Autodesk Fusion 360 part; units mm, degrees
(part 4 of 4)
  spline S343 degree 2 poles (11.0558, -7.1187) (11.2604, -7.2715) (11.3409, -7.5484) knots 0 0 0 1 1 1
  line L153 (11.3409, -7.5484) -> (11.0803, -7.6098)
  spline S344 degree 2 poles (11.0803, -7.6098) (11.0107, -7.3915) (10.8784, -7.292) knots 0 0 0 1 1 1
  spline S345 degree 2 poles (10.8784, -7.292) (10.7461, -7.1924) (10.5455, -7.1924) knots 0 0 0 1 1 1
  spline S346 degree 2 poles (10.5455, -7.1924) (10.315, -7.1924) (10.1594, -7.3029) knots 0 0 0 1 1 1
  spline S347 degree 2 poles (10.1594, -7.3029) (10.0053, -7.4134) (9.9425, -7.6003) knots 0 0 0 1 1 1
  spline S348 degree 2 poles (9.9425, -7.6003) (9.8798, -7.7858) (9.8798, -7.9836) knots 0 0 0 1 1 1
  spline S349 degree 2 poles (9.8798, -7.9836) (9.8798, -8.2387) (9.9534, -8.4297) knots 0 0 0 1 1 1
  spline S350 degree 2 poles (9.9534, -8.4297) (10.0285, -8.6194) (10.1854, -8.7135) knots 0 0 0 1 1 1
  spline S351 degree 2 poles (3.7147, -8.854) (3.5237, -9.0355) (3.2318, -9.0355) knots 0 0 0 1 1 1
  spline S352 degree 2 poles (3.2318, -9.0355) (2.9685, -9.0355) (2.7938, -8.8786) knots 0 0 0 1 1 1
  spline S353 degree 2 poles (2.7938, -8.8786) (2.6206, -8.7217) (2.596, -8.472) knots 0 0 0 1 1 1
  line L154 (2.596, -8.472) -> (2.8416, -8.4393)
  spline S354 degree 2 poles (2.8416, -8.4393) (2.8839, -8.648) (2.9848, -8.7408) knots 0 0 0 1 1 1
  spline S355 degree 2 poles (2.9848, -8.7408) (3.0871, -8.8322) (3.2331, -8.8322) knots 0 0 0 1 1 1
  spline S356 degree 2 poles (3.2331, -8.8322) (3.4064, -8.8322) (3.5251, -8.7121) knots 0 0 0 1 1 1
  spline S357 degree 2 poles (3.5251, -8.7121) (3.6451, -8.5921) (3.6451, -8.4147) knots 0 0 0 1 1 1
  spline S358 degree 2 poles (3.6451, -8.4147) (3.6451, -8.2456) (3.5346, -8.1364) knots 0 0 0 1 1 1
  spline S359 degree 2 poles (3.5346, -8.1364) (3.4241, -8.0259) (3.2536, -8.0259) knots 0 0 0 1 1 1
  spline S360 degree 2 poles (3.2536, -8.0259) (3.184, -8.0259) (3.0803, -8.0532) knots 0 0 0 1 1 1
  line L155 (3.0803, -8.0532) -> (3.1076, -7.8377)
  spline S361 degree 2 poles (3.1076, -7.8377) (3.1322, -7.8404) (3.1472, -7.8404) knots 0 0 0 1 1 1
  spline S362 degree 2 poles (3.1472, -7.8404) (3.3041, -7.8404) (3.4296, -7.7585) knots 0 0 0 1 1 1
  spline S363 degree 2 poles (3.4296, -7.7585) (3.5551, -7.6767) (3.5551, -7.5061) knots 0 0 0 1 1 1
  spline S364 degree 2 poles (3.5551, -7.5061) (3.5551, -7.3711) (3.4637, -7.2824) knots 0 0 0 1 1 1
  spline S365 degree 2 poles (3.4637, -7.2824) (3.3723, -7.1937) (3.2277, -7.1937) knots 0 0 0 1 1 1
  spline S366 degree 2 poles (3.2277, -7.1937) (3.0844, -7.1937) (2.9889, -7.2838) knots 0 0 0 1 1 1
  spline S367 degree 2 poles (2.9889, -7.2838) (2.8934, -7.3738) (2.8661, -7.5539) knots 0 0 0 1 1 1
  line L156 (2.8661, -7.5539) -> (2.6206, -7.5102)
  spline S368 degree 2 poles (2.6206, -7.5102) (2.6656, -7.2633) (2.8252, -7.1282) knots 0 0 0 1 1 1
  spline S369 degree 2 poles (2.8252, -7.1282) (2.9848, -6.9918) (3.2222, -6.9918) knots 0 0 0 1 1 1
  spline S370 degree 2 poles (3.2222, -6.9918) (3.3859, -6.9918) (3.5237, -7.0628) knots 0 0 0 1 1 1
  spline S371 degree 2 poles (3.5237, -7.0628) (3.6615, -7.1323) (3.7338, -7.2538) knots 0 0 0 1 1 1
  spline S372 degree 2 poles (3.7338, -7.2538) (3.8075, -7.3752) (3.8075, -7.5116) knots 0 0 0 1 1 1
  spline S373 degree 2 poles (3.8075, -7.5116) (3.8075, -7.6412) (3.7379, -7.7476) knots 0 0 0 1 1 1
  spline S374 degree 2 poles (3.7379, -7.7476) (3.6683, -7.854) (3.5319, -7.9168) knots 0 0 0 1 1 1
  spline S375 degree 2 poles (3.5319, -7.9168) (3.7092, -7.9577) (3.8075, -8.0873) knots 0 0 0 1 1 1
  spline S376 degree 2 poles (3.8075, -8.0873) (3.9057, -8.2156) (3.9057, -8.4093) knots 0 0 0 1 1 1
  spline S377 degree 2 poles (3.9057, -8.4093) (3.9057, -8.6712) (3.7147, -8.854) knots 0 0 0 1 1 1
  line L157 (-0.0141, -2.5211) -> (-0.2842, -2.5211)
  line L158 (-0.2842, -2.5211) -> (-0.2842, -3)
  line L159 (-0.2842, -3) -> (-0.5298, -3)
  line L160 (-0.5298, -3) -> (-0.5298, -2.5211)
  line L161 (-0.5298, -2.5211) -> (-1.3975, -2.5211)
  line L162 (-1.3975, -2.5211) -> (-1.3975, -2.296)
  line L163 (-1.3975, -2.296) -> (-0.4848, -1)
  line L164 (-0.4848, -1) -> (-0.2842, -1)
  line L165 (-0.2842, -1) -> (-0.2842, -2.296)
  line L166 (-0.2842, -2.296) -> (-0.0141, -2.296)
  line L167 (-0.0141, -2.296) -> (-0.0141, -2.5211)
  line L168 (-5.8463, -2.1528) -> (-5.0919, -2.1528)
  line L169 (-5.0919, -2.1528) -> (-5.0919, -2.3997)
  line L170 (-5.0919, -2.3997) -> (-5.8463, -2.3997)
  line L171 (-5.8463, -2.3997) -> (-5.8463, -2.1528)
  spline S378 degree 2 poles (-2.3822, -4.2592) (-2.228, -4.1214) (-2.1639, -3.9918) knots 0 0 0 1 1 1
  line L172 (-2.1639, -3.9918) -> (-2.0056, -3.9918)
  line L173 (-2.0056, -3.9918) -> (-2.0056, -6)
  line L174 (-2.0056, -6) -> (-2.2512, -6)
  line L175 (-2.2512, -6) -> (-2.2512, -4.4352)
  spline S379 degree 2 poles (-2.2512, -4.4352) (-2.3399, -4.5198) (-2.4845, -4.6044) knots 0 0 0 1 1 1
  spline S380 degree 2 poles (-2.4845, -4.6044) (-2.6277, -4.6889) (-2.7423, -4.7312) knots 0 0 0 1 1 1
  line L176 (-2.7423, -4.7312) -> (-2.7423, -4.4939)
  spline S381 degree 2 poles (-2.7423, -4.4939) (-2.5363, -4.397) (-2.3822, -4.2592) knots 0 0 0 1 1 1
  spline S382 degree 2 poles (-4.2457, -5.9168) (-4.389, -6.0341) (-4.6086, -6.0341) knots 0 0 0 1 1 1
  spline S383 degree 2 poles (-4.6086, -6.0341) (-4.8979, -6.0341) (-5.0629, -5.8267) knots 0 0 0 1 1 1
  spline S384 degree 2 poles (-5.0629, -5.8267) (-5.2607, -5.5771) (-5.2607, -5.0136) knots 0 0 0 1 1 1
  spline S385 degree 2 poles (-5.2607, -5.0136) (-5.2607, -4.6589) (-5.1884, -4.4434) knots 0 0 0 1 1 1
  spline S386 degree 2 poles (-5.1884, -4.4434) (-5.1148, -4.2265) (-4.9715, -4.1091) knots 0 0 0 1 1 1
  spline S387 degree 2 poles (-4.9715, -4.1091) (-4.8269, -3.9918) (-4.6086, -3.9918) knots 0 0 0 1 1 1
  spline S388 degree 2 poles (-4.6086, -3.9918) (-4.4476, -3.9918) (-4.3262, -4.0573) knots 0 0 0 1 1 1
  spline S389 degree 2 poles (-4.3262, -4.0573) (-4.2048, -4.1214) (-4.1257, -4.2442) knots 0 0 0 1 1 1
  spline S390 degree 2 poles (-4.1257, -4.2442) (-4.0466, -4.3656) (-4.0015, -4.5416) knots 0 0 0 1 1 1
  spline S391 degree 2 poles (-4.0015, -4.5416) (-3.9565, -4.7162) (-3.9565, -5.0136) knots 0 0 0 1 1 1
  spline S392 degree 2 poles (-3.9565, -5.0136) (-3.9565, -5.3656) (-4.0288, -5.5825) knots 0 0 0 1 1 1
  spline S393 degree 2 poles (-4.0288, -5.5825) (-4.1011, -5.7981) (-4.2457, -5.9168) knots 0 0 0 1 1 1
  spline S394 degree 2 poles (-7.3165, -0.0412) (-7.4213, -0.1198) (-7.5801, -0.1607) knots 0 0 0 1 1 1
  spline S395 degree 2 poles (-7.5801, -0.1607) (-7.7373, -0.2) (-7.9665, -0.2) knots 0 0 0 1 1 1
  line L177 (-7.9665, -0.2) -> (-8.8816, -0.2)
  line L178 (-8.8816, -0.2) -> (-8.8816, 2.2)
  line L179 (-8.8816, 2.2) -> (-7.9812, 2.2)
  spline S396 degree 2 poles (-7.9812, 2.2) (-7.7062, 2.2) (-7.5408, 2.1263) knots 0 0 0 1 1 1
  spline S397 degree 2 poles (-7.5408, 2.1263) (-7.3738, 2.0543) (-7.2805, 1.902) knots 0 0 0 1 1 1
  spline S398 degree 2 poles (-7.2805, 1.902) (-7.1856, 1.7514) (-7.1856, 1.5861) knots 0 0 0 1 1 1
  spline S399 degree 2 poles (-7.1856, 1.5861) (-7.1856, 1.4322) (-7.2691, 1.2963) knots 0 0 0 1 1 1
  spline S400 degree 2 poles (-7.2691, 1.2963) (-7.3526, 1.1604) (-7.5212, 1.0769) knots 0 0 0 1 1 1
  spline S401 degree 2 poles (-7.5212, 1.0769) (-7.3035, 1.0131) (-7.1872, 0.8592) knots 0 0 0 1 1 1
  spline S402 degree 2 poles (-7.1872, 0.8592) (-7.0693, 0.7053) (-7.0693, 0.4958) knots 0 0 0 1 1 1
  spline S403 degree 2 poles (-7.0693, 0.4958) (-7.0693, 0.3271) (-7.1414, 0.1814) knots 0 0 0 1 1 1
  spline S404 degree 2 poles (-7.1414, 0.1814) (-7.2118, 0.0374) (-7.3165, -0.0412) knots 0 0 0 1 1 1
  spline S405 degree 2 poles (-10.9718, -6.0341) (-11.2433, -6.0341) (-11.4275, -5.955) knots 0 0 0 1 1 1
  spline S406 degree 2 poles (-11.4275, -5.955) (-11.6103, -5.8759) (-11.7153, -5.7176) knots 0 0 0 1 1 1
  spline S407 degree 2 poles (-11.7153, -5.7176) (-11.819, -5.558) (-11.8245, -5.3574) knots 0 0 0 1 1 1
  line L180 (-11.8245, -5.3574) -> (-11.5748, -5.3356)
  spline S408 degree 2 poles (-11.5748, -5.3356) (-11.5571, -5.4857) (-11.493, -5.5825) knots 0 0 0 1 1 1
  spline S409 degree 2 poles (-11.493, -5.5825) (-11.4275, -5.678) (-11.2911, -5.7381) knots 0 0 0 1 1 1
  spline S410 degree 2 poles (-11.2911, -5.7381) (-11.1546, -5.7967) (-10.9841, -5.7967) knots 0 0 0 1 1 1
  spline S411 degree 2 poles (-10.9841, -5.7967) (-10.8327, -5.7967) (-10.7167, -5.7517) knots 0 0 0 1 1 1
  spline S412 degree 2 poles (-10.7167, -5.7517) (-10.6008, -5.7067) (-10.5448, -5.6289) knots 0 0 0 1 1 1
  spline S413 degree 2 poles (-10.5448, -5.6289) (-10.4875, -5.5498) (-10.4875, -5.457) knots 0 0 0 1 1 1
  spline S414 degree 2 poles (-10.4875, -5.457) (-10.4875, -5.3629) (-10.5421, -5.2933) knots 0 0 0 1 1 1
  spline S415 degree 2 poles (-10.5421, -5.2933) (-10.5967, -5.2224) (-10.7222, -5.1746) knots 0 0 0 1 1 1
  spline S416 degree 2 poles (-10.7222, -5.1746) (-10.8027, -5.1432) (-11.0782, -5.0778) knots 0 0 0 1 1 1
  spline S417 degree 2 poles (-11.0782, -5.0778) (-11.3538, -5.0109) (-11.4643, -4.9523) knots 0 0 0 1 1 1
  spline S418 degree 2 poles (-11.4643, -4.9523) (-11.6076, -4.8772) (-11.6785, -4.7667) knots 0 0 0 1 1 1
  spline S419 degree 2 poles (-11.6785, -4.7667) (-11.7481, -4.6548) (-11.7481, -4.5171) knots 0 0 0 1 1 1
  spline S420 degree 2 poles (-11.7481, -4.5171) (-11.7481, -4.3656) (-11.6621, -4.2347) knots 0 0 0 1 1 1
  spline S421 degree 2 poles (-11.6621, -4.2347) (-11.5762, -4.1023) (-11.4111, -4.0341) knots 0 0 0 1 1 1
  spline S422 degree 2 poles (-11.4111, -4.0341) (-11.246, -3.9659) (-11.0441, -3.9659) knots 0 0 0 1 1 1
  spline S423 degree 2 poles (-11.0441, -3.9659) (-10.8218, -3.9659) (-10.6526, -4.0382) knots 0 0 0 1 1 1
  spline S424 degree 2 poles (-10.6526, -4.0382) (-10.4821, -4.1091) (-10.3907, -4.2483) knots 0 0 0 1 1 1
  spline S425 degree 2 poles (-10.3907, -4.2483) (-10.2993, -4.3874) (-10.2924, -4.5634) knots 0 0 0 1 1 1
  line L181 (-10.2924, -4.5634) -> (-10.5462, -4.5825)
  spline S426 degree 2 poles (-10.5462, -4.5825) (-10.5666, -4.3929) (-10.6853, -4.296) knots 0 0 0 1 1 1
  spline S427 degree 2 poles (-10.6853, -4.296) (-10.8027, -4.1992) (-11.0332, -4.1992) knots 0 0 0 1 1 1
  spline S428 degree 2 poles (-11.0332, -4.1992) (-11.2733, -4.1992) (-11.3838, -4.2879) knots 0 0 0 1 1 1
  spline S429 degree 2 poles (-11.3838, -4.2879) (-11.493, -4.3752) (-11.493, -4.4993) knots 0 0 0 1 1 1
  spline S430 degree 2 poles (-11.493, -4.4993) (-11.493, -4.6071) (-11.4152, -4.6767) knots 0 0 0 1 1 1
  spline S431 degree 2 poles (-11.4152, -4.6767) (-11.3388, -4.7462) (-11.0168, -4.8199) knots 0 0 0 1 1 1
  spline S432 degree 2 poles (-11.0168, -4.8199) (-10.6935, -4.8922) (-10.5735, -4.9468) knots 0 0 0 1 1 1
  spline S433 degree 2 poles (-10.5735, -4.9468) (-10.3988, -5.0273) (-10.3156, -5.1514) knots 0 0 0 1 1 1
  spline S434 degree 2 poles (-10.3156, -5.1514) (-10.2324, -5.2742) (-10.2324, -5.4352) knots 0 0 0 1 1 1
  spline S435 degree 2 poles (-10.2324, -5.4352) (-10.2324, -5.5948) (-10.3238, -5.7367) knots 0 0 0 1 1 1
  spline S436 degree 2 poles (-10.3238, -5.7367) (-10.4152, -5.8772) (-10.5871, -5.9563) knots 0 0 0 1 1 1
  spline S437 degree 2 poles (-10.5871, -5.9563) (-10.7576, -6.0341) (-10.9718, -6.0341) knots 0 0 0 1 1 1
  line L182 (-7.1267, -8.1869) -> (-7.6397, -8.1869)
  line L183 (-7.6397, -8.1869) -> (-7.6397, -9)
  line L184 (-7.6397, -9) -> (-7.9043, -9)
  line L185 (-7.9043, -9) -> (-7.9043, -7)
  line L186 (-7.9043, -7) -> (-7.1499, -7)
  spline S438 degree 2 poles (-7.1499, -7) (-6.9507, -7) (-6.8457, -7.0191) knots 0 0 0 1 1 1
  spline S439 degree 2 poles (-6.8457, -7.0191) (-6.6983, -7.0437) (-6.5987, -7.1132) knots 0 0 0 1 1 1
  spline S440 degree 2 poles (-6.5987, -7.1132) (-6.4991, -7.1814) (-6.4391, -7.3056) knots 0 0 0 1 1 1
  spline S441 degree 2 poles (-6.4391, -7.3056) (-6.3777, -7.4297) (-6.3777, -7.5784) knots 0 0 0 1 1 1
  spline S442 degree 2 poles (-6.3777, -7.5784) (-6.3777, -7.8336) (-6.5401, -8.0109) knots 0 0 0 1 1 1
  spline S443 degree 2 poles (-6.5401, -8.0109) (-6.7024, -8.1869) (-7.1267, -8.1869) knots 0 0 0 1 1 1
  spline S444 degree 2 poles (-8.7686, -4.2415) (-8.7999, -4.3793) (-8.8272, -4.4761) knots 0 0 0 1 1 1
  line L187 (-8.8272, -4.4761) -> (-9.2515, -6)
  line L188 (-9.2515, -6) -> (-9.5216, -6)
  line L189 (-9.5216, -6) -> (-10.0523, -4)
  line L190 (-10.0523, -4) -> (-9.7808, -4)
  line L191 (-9.7808, -4) -> (-9.4766, -5.3111)
  spline S445 degree 2 poles (-9.4766, -5.3111) (-9.4275, -5.5171) (-9.392, -5.7203) knots 0 0 0 1 1 1
  spline S446 degree 2 poles (-9.392, -5.7203) (-9.3156, -5.3997) (-9.302, -5.3506) knots 0 0 0 1 1 1
  line L192 (-9.302, -5.3506) -> (-8.9214, -4)
  line L193 (-8.9214, -4) -> (-8.6021, -4)
  line L194 (-8.6021, -4) -> (-8.3156, -5.0123)
  spline S447 degree 2 poles (-8.3156, -5.0123) (-8.2078, -5.3888) (-8.1601, -5.7203) knots 0 0 0 1 1 1
  spline S448 degree 2 poles (-8.1601, -5.7203) (-8.1219, -5.5307) (-8.0605, -5.2851) knots 0 0 0 1 1 1
  line L195 (-8.0605, -5.2851) -> (-7.7467, -4)
  line L196 (-7.7467, -4) -> (-7.4807, -4)
  line L197 (-7.4807, -4) -> (-8.0291, -6)
  line L198 (-8.0291, -6) -> (-8.2842, -6)
  line L199 (-8.2842, -6) -> (-8.7058, -4.4761)
  spline S449 degree 2 poles (-8.7058, -4.4761) (-8.759, -4.2851) (-8.7686, -4.2415) knots 0 0 0 1 1 1
  line L200 (-9.8845, -2.1528) -> (-9.1301, -2.1528)
  line L201 (-9.1301, -2.1528) -> (-9.1301, -2.3997)
  line L202 (-9.1301, -2.3997) -> (-9.8845, -2.3997)
  line L203 (-9.8845, -2.3997) -> (-9.8845, -2.1528)
  line L204 (-3.5691, -5.7203) -> (-3.2894, -5.7203)
  line L205 (-3.2894, -5.7203) -> (-3.2894, -6)
  line L206 (-3.2894, -6) -> (-3.5691, -6)
  line L207 (-3.5691, -6) -> (-3.5691, -5.7203)
  line L208 (-0.1598, -5.3943) -> (-0.9961, -5.3943)
  line L209 (-0.9961, -5.3943) -> (-1.2157, -6)
  line L210 (-1.2157, -6) -> (-1.4968, -6)
  line L211 (-1.4968, -6) -> (-0.7287, -4)
  line L212 (-0.7287, -4) -> (-0.4436, -4)
  line L213 (-0.4436, -4) -> (0.375, -6)
  line L214 (0.375, -6) -> (0.0735, -6)
  line L215 (0.0735, -6) -> (-0.1598, -5.3943)
  spline S450 degree 2 poles (-5.4656, -0.2409) (-5.7914, -0.2409) (-6.0124, -0.146) knots 0 0 0 1 1 1
  spline S451 degree 2 poles (-6.0124, -0.146) (-6.2318, -0.051) (-6.3579, 0.1389) knots 0 0 0 1 1 1
  spline S452 degree 2 poles (-6.3579, 0.1389) (-6.4823, 0.3304) (-6.4888, 0.5711) knots 0 0 0 1 1 1
  line L216 (-6.4888, 0.5711) -> (-6.1892, 0.5973)
  spline S453 degree 2 poles (-6.1892, 0.5973) (-6.168, 0.4172) (-6.091, 0.301) knots 0 0 0 1 1 1
  spline S454 degree 2 poles (-6.091, 0.301) (-6.0124, 0.1864) (-5.8487, 0.1143) knots 0 0 0 1 1 1
  spline S455 degree 2 poles (-5.8487, 0.1143) (-5.685, 0.0439) (-5.4804, 0.0439) knots 0 0 0 1 1 1
  spline S456 degree 2 poles (-5.4804, 0.0439) (-5.2987, 0.0439) (-5.1595, 0.098) knots 0 0 0 1 1 1
  spline S457 degree 2 poles (-5.1595, 0.098) (-5.0203, 0.152) (-4.9532, 0.2453) knots 0 0 0 1 1 1
  spline S458 degree 2 poles (-4.9532, 0.2453) (-4.8845, 0.3402) (-4.8845, 0.4516) knots 0 0 0 1 1 1
  spline S459 degree 2 poles (-4.8845, 0.4516) (-4.8845, 0.5645) (-4.9499, 0.648) knots 0 0 0 1 1 1
  spline S460 degree 2 poles (-4.9499, 0.648) (-5.0154, 0.7332) (-5.166, 0.7905) knots 0 0 0 1 1 1
  spline S461 degree 2 poles (-5.166, 0.7905) (-5.2626, 0.8281) (-5.5933, 0.9067) knots 0 0 0 1 1 1
  spline S462 degree 2 poles (-5.5933, 0.9067) (-5.924, 0.9869) (-6.0566, 1.0573) knots 0 0 0 1 1 1
  spline S463 degree 2 poles (-6.0566, 1.0573) (-6.2285, 1.1473) (-6.3137, 1.2799) knots 0 0 0 1 1 1
  spline S464 degree 2 poles (-6.3137, 1.2799) (-6.3971, 1.4142) (-6.3971, 1.5795) knots 0 0 0 1 1 1
  spline S465 degree 2 poles (-6.3971, 1.5795) (-6.3971, 1.7613) (-6.294, 1.9184) knots 0 0 0 1 1 1
  spline S466 degree 2 poles (-6.294, 1.9184) (-6.1909, 2.0772) (-5.9928, 2.1591) knots 0 0 0 1 1 1
  spline S467 degree 2 poles (-5.9928, 2.1591) (-5.7947, 2.2409) (-5.5524, 2.2409) knots 0 0 0 1 1 1
  spline S468 degree 2 poles (-5.5524, 2.2409) (-5.2856, 2.2409) (-5.0826, 2.1542) knots 0 0 0 1 1 1
  spline S469 degree 2 poles (-5.0826, 2.1542) (-4.8779, 2.069) (-4.7682, 1.902) knots 0 0 0 1 1 1
  spline S470 degree 2 poles (-4.7682, 1.902) (-4.6585, 1.7351) (-4.6504, 1.5239) knots 0 0 0 1 1 1
  line L217 (-4.6504, 1.5239) -> (-4.9549, 1.501)
  spline S471 degree 2 poles (-4.9549, 1.501) (-4.9794, 1.7285) (-5.1218, 1.8447) knots 0 0 0 1 1 1
  spline S472 degree 2 poles (-5.1218, 1.8447) (-5.2626, 1.961) (-5.5393, 1.961) knots 0 0 0 1 1 1
  spline S473 degree 2 poles (-5.5393, 1.961) (-5.8274, 1.961) (-5.96, 1.8546) knots 0 0 0 1 1 1
  spline S474 degree 2 poles (-5.96, 1.8546) (-6.091, 1.7498) (-6.091, 1.6008) knots 0 0 0 1 1 1
  spline S475 degree 2 poles (-6.091, 1.6008) (-6.091, 1.4715) (-5.9977, 1.388) knots 0 0 0 1 1 1
  spline S476 degree 2 poles (-5.9977, 1.388) (-5.906, 1.3045) (-5.5197, 1.2161) knots 0 0 0 1 1 1
  spline S477 degree 2 poles (-5.5197, 1.2161) (-5.1317, 1.1293) (-4.9876, 1.0638) knots 0 0 0 1 1 1
  spline S478 degree 2 poles (-4.9876, 1.0638) (-4.778, 0.9673) (-4.6782, 0.8183) knots 0 0 0 1 1 1
  spline S479 degree 2 poles (-4.6782, 0.8183) (-4.5783, 0.6709) (-4.5783, 0.4778) knots 0 0 0 1 1 1
  spline S480 degree 2 poles (-4.5783, 0.4778) (-4.5783, 0.2862) (-4.688, 0.116) knots 0 0 0 1 1 1
  spline S481 degree 2 poles (-4.688, 0.116) (-4.7977, -0.0527) (-5.004, -0.1476) knots 0 0 0 1 1 1
  spline S482 degree 2 poles (-5.004, -0.1476) (-5.2086, -0.2409) (-5.4656, -0.2409) knots 0 0 0 1 1 1
  line L218 (7.1581, -4) -> (7.4282, -4)
  line L219 (7.4282, -4) -> (6.6451, -6)
  line L220 (6.6451, -6) -> (6.3736, -6)
  line L221 (6.3736, -6) -> (5.5987, -4)
  line L222 (5.5987, -4) -> (5.8852, -4)
  line L223 (5.8852, -4) -> (6.405, -5.4529)
  spline S483 degree 2 poles (6.405, -5.4529) (6.4678, -5.6276) (6.5101, -5.7804) knots 0 0 0 1 1 1
  spline S484 degree 2 poles (6.5101, -5.7804) (6.5564, -5.6166) (6.6178, -5.4529) knots 0 0 0 1 1 1
  line L224 (6.6178, -5.4529) -> (7.1581, -4)
  spline S485 degree 2 poles (5.1635, -8.9168) (5.0203, -9.0341) (4.8006, -9.0341) knots 0 0 0 1 1 1
  spline S486 degree 2 poles (4.8006, -9.0341) (4.5114, -9.0341) (4.3464, -8.8267) knots 0 0 0 1 1 1
  spline S487 degree 2 poles (4.3464, -8.8267) (4.1485, -8.5771) (4.1485, -8.0136) knots 0 0 0 1 1 1
  spline S488 degree 2 poles (4.1485, -8.0136) (4.1485, -7.6589) (4.2208, -7.4434) knots 0 0 0 1 1 1
  spline S489 degree 2 poles (4.2208, -7.4434) (4.2945, -7.2265) (4.4378, -7.1091) knots 0 0 0 1 1 1
  spline S490 degree 2 poles (4.4378, -7.1091) (4.5824, -6.9918) (4.8006, -6.9918) knots 0 0 0 1 1 1
  spline S491 degree 2 poles (4.8006, -6.9918) (4.9616, -6.9918) (5.083, -7.0573) knots 0 0 0 1 1 1
  spline S492 degree 2 poles (5.083, -7.0573) (5.2045, -7.1214) (5.2836, -7.2442) knots 0 0 0 1 1 1
  spline S493 degree 2 poles (5.2836, -7.2442) (5.3627, -7.3656) (5.4077, -7.5416) knots 0 0 0 1 1 1
  spline S494 degree 2 poles (5.4077, -7.5416) (5.4528, -7.7162) (5.4528, -8.0136) knots 0 0 0 1 1 1
  spline S495 degree 2 poles (5.4528, -8.0136) (5.4528, -8.3656) (5.3805, -8.5825) knots 0 0 0 1 1 1
  spline S496 degree 2 poles (5.3805, -8.5825) (5.3082, -8.7981) (5.1635, -8.9168) knots 0 0 0 1 1 1
  spline S497 degree 2 poles (10.1854, -5.7135) (10.3423, -5.8076) (10.5251, -5.8076) knots 0 0 0 1 1 1
  spline S498 degree 2 poles (10.5251, -5.8076) (10.7474, -5.8076) (10.9016, -5.6794) knots 0 0 0 1 1 1
  spline S499 degree 2 poles (10.9016, -5.6794) (11.0558, -5.5512) (11.1103, -5.2988) knots 0 0 0 1 1 1
  line L225 (11.1103, -5.2988) -> (11.375, -5.3656)
  spline S500 degree 2 poles (11.375, -5.3656) (11.2918, -5.6917) (11.0749, -5.8636) knots 0 0 0 1 1 1
  spline S501 degree 2 poles (11.0749, -5.8636) (10.8593, -6.0341) (10.5469, -6.0341) knots 0 0 0 1 1 1
  spline S502 degree 2 poles (10.5469, -6.0341) (10.2236, -6.0341) (10.0203, -5.9031) knots 0 0 0 1 1 1
  spline S503 degree 2 poles (10.0203, -5.9031) (9.8184, -5.7708) (9.712, -5.5211) knots 0 0 0 1 1 1
  spline S504 degree 2 poles (9.712, -5.5211) (9.6069, -5.2715) (9.6069, -4.985) knots 0 0 0 1 1 1
  spline S505 degree 2 poles (9.6069, -4.985) (9.6069, -4.6726) (9.7256, -4.4407) knots 0 0 0 1 1 1
  spline S506 degree 2 poles (9.7256, -4.4407) (9.8457, -4.2074) (10.0653, -4.0873) knots 0 0 0 1 1 1
  spline S507 degree 2 poles (10.0653, -4.0873) (10.2863, -3.9659) (10.551, -3.9659) knots 0 0 0 1 1 1
  spline S508 degree 2 poles (10.551, -3.9659) (10.8511, -3.9659) (11.0558, -4.1187) knots 0 0 0 1 1 1
  spline S509 degree 2 poles (11.0558, -4.1187) (11.2604, -4.2715) (11.3409, -4.5484) knots 0 0 0 1 1 1
  line L226 (11.3409, -4.5484) -> (11.0803, -4.6098)
  spline S510 degree 2 poles (11.0803, -4.6098) (11.0107, -4.3915) (10.8784, -4.292) knots 0 0 0 1 1 1
  spline S511 degree 2 poles (10.8784, -4.292) (10.7461, -4.1924) (10.5455, -4.1924) knots 0 0 0 1 1 1
  spline S512 degree 2 poles (10.5455, -4.1924) (10.315, -4.1924) (10.1594, -4.3029) knots 0 0 0 1 1 1
  spline S513 degree 2 poles (10.1594, -4.3029) (10.0053, -4.4134) (9.9425, -4.6003) knots 0 0 0 1 1 1
  spline S514 degree 2 poles (9.9425, -4.6003) (9.8798, -4.7858) (9.8798, -4.9836) knots 0 0 0 1 1 1
  spline S515 degree 2 poles (9.8798, -4.9836) (9.8798, -5.2387) (9.9534, -5.4297) knots 0 0 0 1 1 1
  spline S516 degree 2 poles (9.9534, -5.4297) (10.0285, -5.6194) (10.1854, -5.7135) knots 0 0 0 1 1 1
  spline S517 degree 2 poles (6.5275, -1.2592) (6.6816, -1.1214) (6.7458, -0.9918) knots 0 0 0 1 1 1
  line L227 (6.7458, -0.9918) -> (6.904, -0.9918)
  line L228 (6.904, -0.9918) -> (6.904, -3)
  line L229 (6.904, -3) -> (6.6585, -3)
  line L230 (6.6585, -3) -> (6.6585, -1.4352)
  spline S518 degree 2 poles (6.6585, -1.4352) (6.5698, -1.5198) (6.4252, -1.6044) knots 0 0 0 1 1 1
  spline S519 degree 2 poles (6.4252, -1.6044) (6.2819, -1.6889) (6.1673, -1.7312) knots 0 0 0 1 1 1
  line L231 (6.1673, -1.7312) -> (6.1673, -1.4939)
  spline S520 degree 2 poles (6.1673, -1.4939) (6.3733, -1.397) (6.5275, -1.2592) knots 0 0 0 1 1 1
  line L232 (0.2096, -2.1528) -> (0.964, -2.1528)
  line L233 (0.964, -2.1528) -> (0.964, -2.3997)
  line L234 (0.964, -2.3997) -> (0.2096, -2.3997)
  line L235 (0.2096, -2.3997) -> (0.2096, -2.1528)
  spline S521 degree 2 poles (7.7779, 1.8889) (7.9629, 2.0543) (8.0398, 2.2098) knots 0 0 0 1 1 1
  line L236 (8.0398, 2.2098) -> (8.2298, 2.2098)
  line L237 (8.2298, 2.2098) -> (8.2298, -0.2)
  line L238 (8.2298, -0.2) -> (7.9351, -0.2)
  line L239 (7.9351, -0.2) -> (7.9351, 1.6778)
  spline S522 degree 2 poles (7.9351, 1.6778) (7.8287, 1.5763) (7.6551, 1.4748) knots 0 0 0 1 1 1
  spline S523 degree 2 poles (7.6551, 1.4748) (7.4832, 1.3733) (7.3457, 1.3225) knots 0 0 0 1 1 1
  line L240 (7.3457, 1.3225) -> (7.3457, 1.6074)
  spline S524 degree 2 poles (7.3457, 1.6074) (7.5929, 1.7236) (7.7779, 1.8889) knots 0 0 0 1 1 1
  spline S525 degree 2 poles (-9.2484, 3.3595) (-9.3917, 3.2234) (-9.6106, 3.2234) knots 0 0 0 1 1 1
  spline S526 degree 2 poles (-9.6106, 3.2234) (-9.8081, 3.2234) (-9.9391, 3.3411) knots 0 0 0 1 1 1
  spline S527 degree 2 poles (-9.9391, 3.3411) (-10.069, 3.4587) (-10.0875, 3.646) knots 0 0 0 1 1 1
  line L241 (-10.0875, 3.646) -> (-9.9033, 3.6705)
  spline S528 degree 2 poles (-9.9033, 3.6705) (-9.8716, 3.514) (-9.7958, 3.4444) knots 0 0 0 1 1 1
  spline S529 degree 2 poles (-9.7958, 3.4444) (-9.7191, 3.3759) (-9.6096, 3.3759) knots 0 0 0 1 1 1
  spline S530 degree 2 poles (-9.6096, 3.3759) (-9.4797, 3.3759) (-9.3907, 3.4659) knots 0 0 0 1 1 1
  spline S531 degree 2 poles (-9.3907, 3.4659) (-9.3006, 3.5559) (-9.3006, 3.6889) knots 0 0 0 1 1 1
  spline S532 degree 2 poles (-9.3006, 3.6889) (-9.3006, 3.8158) (-9.3835, 3.8977) knots 0 0 0 1 1 1
  spline S533 degree 2 poles (-9.3835, 3.8977) (-9.4664, 3.9806) (-9.5943, 3.9806) knots 0 0 0 1 1 1
  spline S534 degree 2 poles (-9.5943, 3.9806) (-9.6465, 3.9806) (-9.7242, 3.9601) knots 0 0 0 1 1 1
  line L242 (-9.7242, 3.9601) -> (-9.7038, 4.1218)
  spline S535 degree 2 poles (-9.7038, 4.1218) (-9.6853, 4.1197) (-9.6741, 4.1197) knots 0 0 0 1 1 1
  spline S536 degree 2 poles (-9.6741, 4.1197) (-9.5564, 4.1197) (-9.4623, 4.1811) knots 0 0 0 1 1 1
  spline S537 degree 2 poles (-9.4623, 4.1811) (-9.3681, 4.2425) (-9.3681, 4.3704) knots 0 0 0 1 1 1
  spline S538 degree 2 poles (-9.3681, 4.3704) (-9.3681, 4.4717) (-9.4367, 4.5382) knots 0 0 0 1 1 1
  spline S539 degree 2 poles (-9.4367, 4.5382) (-9.5053, 4.6047) (-9.6137, 4.6047) knots 0 0 0 1 1 1
  spline S540 degree 2 poles (-9.6137, 4.6047) (-9.7211, 4.6047) (-9.7928, 4.5372) knots 0 0 0 1 1 1
  spline S541 degree 2 poles (-9.7928, 4.5372) (-9.8644, 4.4696) (-9.8849, 4.3346) knots 0 0 0 1 1 1
  line L243 (-9.8849, 4.3346) -> (-10.069, 4.3673)
  spline S542 degree 2 poles (-10.069, 4.3673) (-10.0353, 4.5525) (-9.9156, 4.6538) knots 0 0 0 1 1 1
  spline S543 degree 2 poles (-9.9156, 4.6538) (-9.7958, 4.7561) (-9.6178, 4.7561) knots 0 0 0 1 1 1
  spline S544 degree 2 poles (-9.6178, 4.7561) (-9.495, 4.7561) (-9.3917, 4.7029) knots 0 0 0 1 1 1
  spline S545 degree 2 poles (-9.3917, 4.7029) (-9.2883, 4.6508) (-9.2341, 4.5597) knots 0 0 0 1 1 1
  spline S546 degree 2 poles (-9.2341, 4.5597) (-9.1789, 4.4686) (-9.1789, 4.3663) knots 0 0 0 1 1 1
  spline S547 degree 2 poles (-9.1789, 4.3663) (-9.1789, 4.2691) (-9.231, 4.1893) knots 0 0 0 1 1 1
  spline S548 degree 2 poles (-9.231, 4.1893) (-9.2832, 4.1095) (-9.3855, 4.0624) knots 0 0 0 1 1 1
  spline S549 degree 2 poles (-9.3855, 4.0624) (-9.2525, 4.0317) (-9.1789, 3.9345) knots 0 0 0 1 1 1
  spline S550 degree 2 poles (-9.1789, 3.9345) (-9.1052, 3.8383) (-9.1052, 3.693) knots 0 0 0 1 1 1
  spline S551 degree 2 poles (-9.1052, 3.693) (-9.1052, 3.4966) (-9.2484, 3.3595) knots 0 0 0 1 1 1
  line L244 (-4.0281, 3.25) -> (-4.816, 4.4287)
  line L245 (-4.816, 4.4287) -> (-4.816, 3.25)
  line L246 (-4.816, 3.25) -> (-5.0063, 3.25)
  line L247 (-5.0063, 3.25) -> (-5.0063, 4.75)
  line L248 (-5.0063, 4.75) -> (-4.8027, 4.75)
  line L249 (-4.8027, 4.75) -> (-4.0148, 3.5723)
  line L250 (-4.0148, 3.5723) -> (-4.0148, 4.75)
  line L251 (-4.0148, 4.75) -> (-3.8245, 4.75)
  line L252 (-3.8245, 4.75) -> (-3.8245, 3.25)
  line L253 (-3.8245, 3.25) -> (-4.0281, 3.25)
  line L254 (-15.3245, 10.25) -> (-15.3245, 11.25)
  line L255 (-15.3245, 11.25) -> (-19.375, 11.25)
  arc A0 (-19.375, 11.25) -> (-21.8245, 9.25) centre (-19.375, 8.75) ccw
  line L256 (-21.8245, 9.25) -> (-21.875, -5.25)
  line L257 (-21.875, -5.25) -> (-21.875, -6.25)
  arc A1 (-21.875, -6.25) -> (-16.875, -11.25) centre (-16.875, -6.25) ccw
  line L258 (-16.875, -11.25) -> (-16.8245, -11.25)
  line L259 (-16.8245, -11.25) -> (-16.8245, -10.25)
  line L260 (-16.8245, -10.25) -> (-13.3245, -10.25)
  line L261 (-13.3245, -10.25) -> (-13.3245, -11.25)
  line L262 (-13.3245, -11.25) -> (0.275, -11.25)
  arc A2 (0.275, -11.25) -> (8.375, -11.25) centre (4.325, -9.2195) ccw
  line L263 (8.375, -11.25) -> (16.875, -11.25)
  arc A3 (16.875, -11.25) -> (21.875, -6.25) centre (16.875, -6.25) ccw
  line L264 (21.875, -6.25) -> (21.875, -1)
  line L265 (21.875, -1) -> (20.875, -1)
  line L266 (20.875, -1) -> (20.875, 1)
  line L267 (20.875, 1) -> (21.875, 1)
  line L268 (21.875, 1) -> (21.875, 2.5)
  line L269 (21.875, 2.5) -> (21.875, 8.75)
  arc A4 (21.875, 8.75) -> (19.375, 11.25) centre (19.375, 8.75) ccw
  line L270 (19.375, 11.25) -> (6.875, 11.25)
  line L271 (6.875, 11.25) -> (6.875, 6.75)
  line L272 (6.875, 6.75) -> (-7.8245, 6.75)
  line L273 (-7.8245, 6.75) -> (-7.8245, 11.25)
  line L274 (-7.8245, 11.25) -> (-13.3245, 11.25)
  line L275 (-13.3245, 11.25) -> (-13.3245, 10.25)
  line L276 (-13.3245, 10.25) -> (-15.3245, 10.25)
  line L277 (6.875, 11.25) -> (1.875, 11.25)
  line L278 (1.875, 11.25) -> (1.875, 6.75)
  line L279 (1.875, 6.75) -> (6.875, 6.75)
  line L280 (6.875, 6.75) -> (6.875, 11.25)
  line L281 (1.875, 9.25) -> (-7.8245, 9.25)
  line L282 (-7.8245, 9.25) -> (-7.8245, 6.75)
  line L283 (-7.8245, 6.75) -> (1.875, 6.75)
  line L284 (1.875, 6.75) -> (1.875, 9.25)
  dimension "d97" = 5
  dimension "d98" = 2
  constraint horizontal L277
  constraint vertical L278
  constraint horizontal L279
  constraint vertical L280
  constraint coincident L272 L278.end
  constraint coincident L270.end L271.start
  constraint horizontal L281
  constraint vertical L282
  constraint horizontal L283
  constraint vertical L284
  constraint coincident L272.end L273.start
  constraint coincident L278 L281.start
  measures "d97" distance of L270.end L277.end
  measures "d98" distance of L277 L281
extrude "Extrude10" cut sketch "Sketch6" against normal blind 13 contours L272 L273 L278 L281 L282 L283 L284 | L271 L272 L277 L278 L279 L280 L284 in component "housing"
sketch "Sketch7" plane through (13.8245, 0, 0) normal (1, 0, 0) x (0, 1, 0) in component "housing"
  line L0 (-4, -5.25) -> (4, -5.25)
  line L1 (4, -5.25) -> (4, 8.25)
  line L2 (4, 8.25) -> (-8, 8.25)
  line L3 (-8, 8.25) -> (-8, -4.75)
  line L4 (-8, -4.75) -> (-4, -4.75)
  line L5 (-4, -4.75) -> (-4, -5.25)
  line L6 (4, -5.25) -> (-4, -5.25)
  line L7 (-4, -5.25) -> (-4, 8.25)
  line L8 (-4, 8.25) -> (4, 8.25)
  line L9 (4, 8.25) -> (4, -5.25)
  constraint horizontal L6
  constraint vertical L7
  constraint horizontal L8
  constraint vertical L9
  constraint coincident L2 L7.end
  constraint coincident L0.end L1.start
  constraint collinear L5 L7
extrude "Extrude11" cut sketch "Sketch7" against normal blind 33 contours L0 L1 L2 L5 L6 L7 L8 L9 in component "housing"
component "housing" placed x (1, 0, 0) y (0, 1, 0) z (0, 0, 1) at (0, 0, 0)
equation "fillet_radius = 5 mm"
equation "d13 = fillet_radius"
equation "d14 = fillet_radius"
equation "d44 = 15 mm + ( 1.75 * 2 ) * 1 mm"
equation "d48 = 12 mm - 1.5 mm"
equation "d58 = 45 deg + 90 deg"

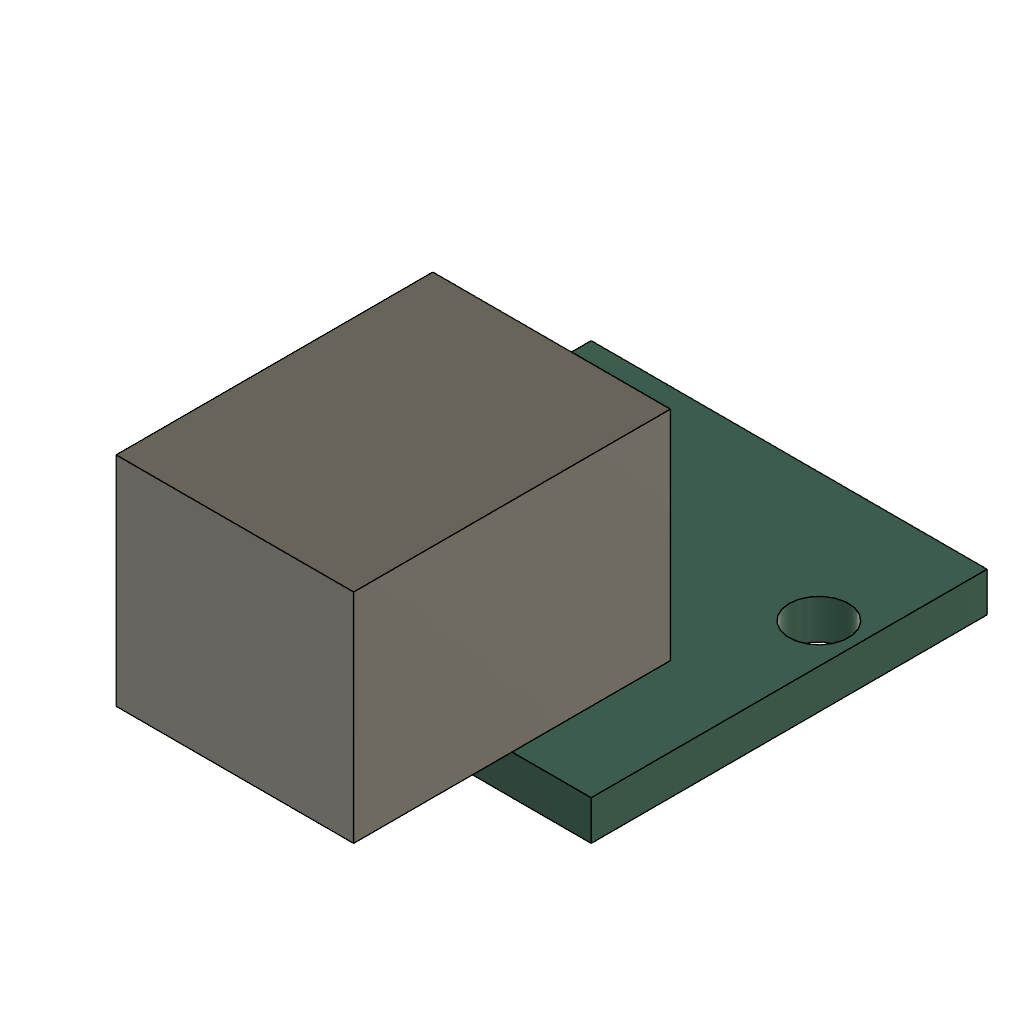
design "usbmodule"
Autodesk Fusion 360 part; units mm, degrees
sketch "Sketch1" plane through (0, 0, 0) normal (0, 0, 1) x (1, 0, 0)
  line L0 (0, 0) -> (20, 0)
  line L1 (20, 0) -> (20, 20)
  line L2 (20, 20) -> (0, 20)
  line L3 (0, 20) -> (0, 0)
  line L4 (4, 8) -> (16, 8)
  line L5 (16, 8) -> (16, -8)
  line L6 (16, -8) -> (4, -8)
  line L7 (4, -8) -> (4, 8)
  line L8 (4, 8) -> (16, -8) construction
  line L9 (16, 8) -> (4, -8) construction
  line L10 (20, 20) -> (0, 20)
  line L11 (0, 20) -> (0, 13.5)
  line L12 (0, 13.5) -> (20, 13.5)
  line L13 (20, 13.5) -> (20, 20)
  line L14 (0, 20) -> (2, 20)
  line L15 (2, 20) -> (2, 13.5)
  line L16 (2, 13.5) -> (0, 13.5)
  line L17 (0, 13.5) -> (0, 20)
  line L18 (20, 20) -> (18, 20)
  line L19 (18, 20) -> (18, 13.5)
  line L20 (18, 13.5) -> (20, 13.5)
  line L21 (20, 13.5) -> (20, 20)
  circle A0 centre (2, 13.5) radius 1.5
  circle A1 centre (18, 13.5) radius 1.5
  point P0 (10, 0)
  dimension "d1" = 20
  dimension "d2" = 20
  dimension "d3" = 16
  dimension "d4" = 20
  dimension "d5" = 6.5
  dimension "d6" = 2
  dimension "d7" = 2
  constraint horizontal L0
  constraint vertical L1
  constraint horizontal L2
  constraint vertical L3
  constraint coincident L0.start L3.end
  constraint horizontal L4
  constraint perpendicular L4 L5
  constraint parallel L4 L6
  constraint parallel L5 L7
  constraint coincident L8 P0
  constraint coincident L9 P0
  constraint midpoint L0 P0
  constraint horizontal L10
  constraint vertical L11
  constraint horizontal L12
  constraint vertical L13
  constraint horizontal L14
  constraint vertical L15
  constraint horizontal L16
  constraint vertical L17
  constraint horizontal L18
  constraint vertical L19
  constraint horizontal L20
  constraint vertical L21
  constraint coincident L15.end L16.start
  constraint coincident L19.end L20.start
  measures "d1" distance of L0.start L0.end
  measures "d2" distance of L0.start L2.end
  measures "d3" distance of L4.end L5.end
  measures "d4" distance of L1.end L2.end
  measures "d5" distance of L1.end L12.end
  measures "d6" distance of L2.end L14.end
  measures "d7" distance of L1.end L18.end
extrude "Extrude1" add sketch "Sketch1" against normal blind 2 contours L0 L1 L3 L4 L5 L7 L12 L16 L20 A0 A1 | L0 L4 L5 L7 | L2 L3 L10 L11 L12 L14 L15 L16 L17 A0 | L2 L10 L12 L15 L19 A0 A1 | L1 L2 L10 L12 L13 L18 L19 L20 L21 A1
extrude "Extrude2" add sketch "Sketch1" along normal blind 11 contours L0 L4 L5 L7 | L0 L5 L6 L7
